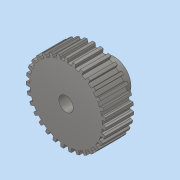
# Autodesk Inventor part: PinionGear
Saved by Autodesk Inventor 2017 (Build 210142000, 142)
## iProperties
Created: 2016-11-06
Part Number: PinionGear
Material: Stainless Steel, Brushed
Document SubType Name: Modeling
Designer: techn
Density: 8 g/cm^3
Appearance: Stainless - Brushed
Author: techn
Comments: 31 Tooth Traxxas Pinion Gear
Autodesk Inventor part; units mm, degrees
ref_plane "YZ Plane" through (0, 0, 0) normal (1, 0, 0) x (0, 1, 0)
ref_plane "XZ Plane" through (0, 0, 0) normal (0, 1, 0) x (-1, 0, 0)
ref_plane "XY Plane" through (0, 0, 0) normal (0, 0, 1) x (1, 0, 0)
sketch "Sketch1" plane through (0, 0, 0) normal (0, 0, 1) x (1, 0, 0)
  circle A0 centre (0, 0) radius 3.7465
  dimension "d0" = 7.493
  constraints: 1 centre point, 1 coincident
  measures "d0" diameter of A0
extrude "Extrusion1" add sketch "Sketch1" along normal blind 10.5156
sketch "Sketch2" plane through (0, 0, 10.5156) normal (0, 0, 1) x (1, 0, 0)
  circle A0 centre (0, 0) radius 8.763
  dimension "d3" = 17.526
  constraints: 1 centre point, 1 coincident
  measures "d3" diameter of A0
extrude "Extrusion2" add sketch "Sketch2" against normal blind 6.096
sketch "Sketch4" plane through (0, 0, 10.5156) normal (0, 0, 1) x (1, 0, 0)
  circle A0 centre (0, 0) radius 1.5875
  dimension "d6" = 3.175
  constraints: 1 centre point, 1 coincident
  measures "d6" diameter of A0
extrude "Extrusion3" cut sketch "Sketch4" against normal through all
sketch "Sketch5" plane through (0, 0, 10.5156) normal (0, 0, 1) x (1, 0, 0)
  circle A0 centre (0, 0) radius 7.9375
  line L0 (0.3683, 7.929) -> (0.3683, 8.31)
  line L1 (0.3683, 8.31) -> (0.2857, 8.89)
  line L2 (0.2857, 8.89) -> (-0.2858, 8.89)
  line L3 (-0.2858, 8.89) -> (-0.3683, 8.31)
  line L4 (-0.3683, 8.31) -> (-0.3683, 7.929)
  line L5 (-0.3683, 7.929) -> (0.3683, 7.929)
  line L6 (-2.0335, 8.0657) -> (-1.9568, 7.6925)
  line L7 (-2.0694, 8.6505) -> (-2.0335, 8.0657)
  line L8 (-1.5096, 8.7655) -> (-2.0694, 8.6505)
  line L9 (-1.312, 8.214) -> (-1.5096, 8.7655)
  line L10 (-1.2353, 7.8408) -> (-1.312, 8.214)
  line L11 (-1.9568, 7.6925) -> (-1.2353, 7.8408)
  line L12 (-3.6155, 7.4913) -> (-3.4653, 7.1411)
  line L13 (-3.7684, 8.0568) -> (-3.6155, 7.4913)
  line L14 (-3.2432, 8.2822) -> (-3.7684, 8.0568)
  line L15 (-2.9386, 7.7817) -> (-3.2432, 8.2822)
  line L16 (-2.7884, 7.4316) -> (-2.9386, 7.7817)
  line L17 (-3.4653, 7.1411) -> (-2.7884, 7.4316)
  line L18 (-5.0495, 6.6101) -> (-4.8318, 6.2974)
  line L19 (-5.3131, 7.1333) -> (-5.0495, 6.6101)
  line L20 (-4.844, 7.4598) -> (-5.3131, 7.1333)
  line L21 (-4.4449, 7.0309) -> (-4.844, 7.4598)
  line L22 (-4.2273, 6.7182) -> (-4.4449, 7.0309)
  line L23 (-4.8318, 6.2974) -> (-4.2273, 6.7182)
  line L24 (-6.2767, 5.4583) -> (-6.0006, 5.1958)
  line L25 (-6.6403, 5.9178) -> (-6.2767, 5.4583)
  line L26 (-6.2465, 6.332) -> (-6.6403, 5.9178)
  line L27 (-5.7692, 5.9922) -> (-6.2465, 6.332)
  line L28 (-5.4931, 5.7297) -> (-5.7692, 5.9922)
  line L29 (-6.0006, 5.1958) -> (-5.4931, 5.7297)
  line L30 (-7.247, 4.0831) -> (-6.9237, 3.8816)
  line L31 (-7.6956, 4.46) -> (-7.247, 4.0831)
  line L32 (-7.3933, 4.945) -> (-7.6956, 4.46)
  line L33 (-6.8574, 4.7082) -> (-7.3933, 4.945)
  line L34 (-6.534, 4.5067) -> (-6.8574, 4.7082)
  line L35 (-6.9237, 3.8816) -> (-6.534, 4.5067)
  line L36 (-7.9206, 2.5407) -> (-7.5633, 2.4084)
  line L37 (-8.4359, 2.8196) -> (-7.9206, 2.5407)
  line L38 (-8.2374, 3.3555) -> (-8.4359, 2.8196)
  line L39 (-7.6648, 3.2315) -> (-8.2374, 3.3555)
  line L40 (-7.3075, 3.0991) -> (-7.6648, 3.2315)
  line L41 (-7.5633, 2.4084) -> (-7.3075, 3.0991)
  line L42 (-8.2699, 0.8943) -> (-7.8933, 0.8366)
  line L43 (-8.8308, 1.0637) -> (-8.2699, 0.8943)
  line L44 (-8.7442, 1.6286) -> (-8.8308, 1.0637)
  line L45 (-8.1584, 1.6224) -> (-8.7442, 1.6286)
  line L46 (-7.7817, 1.5647) -> (-8.1584, 1.6224)
  line L47 (-7.8933, 0.8366) -> (-7.7817, 1.5647)
  line L48 (-8.2806, -0.7887) -> (-7.9001, -0.7694)
  line L49 (-8.8641, -0.7357) -> (-8.2806, -0.7887)
  line L50 (-8.8931, -0.1649) -> (-8.8641, -0.7357)
  line L51 (-8.3179, -0.0531) -> (-8.8931, -0.1649)
  line L52 (-7.9374, -0.0338) -> (-8.3179, -0.0531)
  line L53 (-7.9001, -0.7694) -> (-7.9374, -0.0338)
  line L54 (-7.9524, -2.4395) -> (-7.5835, -2.344)
  line L55 (-8.5346, -2.5049) -> (-7.9524, -2.4395)
  line L56 (-8.6778, -1.9517) -> (-8.5346, -2.5049)
  line L57 (-8.137, -1.7264) -> (-8.6778, -1.9517)
  line L58 (-7.7682, -1.6309) -> (-8.137, -1.7264)
  line L59 (-7.5835, -2.344) -> (-7.7682, -1.6309)
  line L60 (-7.2985, -3.9903) -> (-6.9565, -3.8225)
  line L61 (-7.8556, -4.1717) -> (-7.2985, -3.9903)
  line L62 (-8.1073, -3.6586) -> (-7.8556, -4.1717)
  line L63 (-7.6229, -3.329) -> (-8.1073, -3.6586)
  line L64 (-7.2808, -3.1612) -> (-7.6229, -3.329)
  line L65 (-6.9565, -3.8225) -> (-7.2808, -3.1612)
  line L66 (-6.3459, -5.3778) -> (-6.0446, -5.1446)
  line L67 (-6.8551, -5.6676) -> (-6.3459, -5.3778)
  line L68 (-7.2049, -5.2157) -> (-6.8551, -5.6676)
  line L69 (-6.7967, -4.7953) -> (-7.2049, -5.2157)
  line L70 (-6.4955, -4.5621) -> (-6.7967, -4.7953)
  line L71 (-6.0446, -5.1446) -> (-6.4955, -4.5621)
  line L72 (-5.1334, -6.5451) -> (-4.8852, -6.2561)
  line L73 (-5.5739, -6.9315) -> (-5.1334, -6.5451)
  line L74 (-6.0075, -6.5592) -> (-5.5739, -6.9315)
  line L75 (-5.6923, -6.0653) -> (-6.0075, -6.5592)
  line L76 (-5.4442, -5.7763) -> (-5.6923, -6.0653)
  line L77 (-4.8852, -6.2561) -> (-5.4442, -5.7763)
  line L78 (-3.7108, -7.4445) -> (-3.5259, -7.1114)
  line L79 (-4.0645, -7.9116) -> (-3.7108, -7.4445)
  line L80 (-4.5642, -7.6343) -> (-4.0645, -7.9116)
  line L81 (-4.3549, -7.087) -> (-4.5642, -7.6343)
  line L82 (-4.17, -6.7539) -> (-4.3549, -7.087)
  line L83 (-3.5259, -7.1114) -> (-4.17, -6.7539)
  line L84 (-2.1363, -8.0391) -> (-2.0222, -7.6756)
  line L85 (-2.3887, -8.5678) -> (-2.1363, -8.0391)
  line L86 (-2.934, -8.3968) -> (-2.3887, -8.5678)
  line L87 (-2.8391, -7.8186) -> (-2.934, -8.3968)
  line L88 (-2.725, -7.4551) -> (-2.8391, -7.8186)
  line L89 (-2.0222, -7.6756) -> (-2.725, -7.4551)
  line L90 (-0.4743, -8.3046) -> (-0.4357, -7.9255)
  line L91 (-0.6151, -8.8733) -> (-0.4743, -8.3046)
  line L92 (-1.1837, -8.8155) -> (-0.6151, -8.8733)
  line L93 (-1.2071, -8.2301) -> (-1.1837, -8.8155)
  line L94 (-1.1686, -7.851) -> (-1.2071, -8.2301)
  line L95 (-0.4357, -7.9255) -> (-1.1686, -7.851)
  line L96 (1.2071, -8.2301) -> (1.1686, -7.851)
  line L97 (1.1837, -8.8155) -> (1.2071, -8.2301)
  line L98 (0.6151, -8.8733) -> (1.1837, -8.8155)
  line L99 (0.4743, -8.3046) -> (0.6151, -8.8733)
  line L100 (0.4357, -7.9255) -> (0.4743, -8.3046)
  line L101 (1.1686, -7.851) -> (0.4357, -7.9255)
  line L102 (2.8391, -7.8186) -> (2.725, -7.4551)
  line L103 (2.934, -8.3968) -> (2.8391, -7.8186)
  line L104 (2.3887, -8.5678) -> (2.934, -8.3968)
  line L105 (2.1363, -8.0391) -> (2.3887, -8.5678)
  line L106 (2.0222, -7.6756) -> (2.1363, -8.0391)
  line L107 (2.725, -7.4551) -> (2.0222, -7.6756)
  line L108 (4.3549, -7.087) -> (4.17, -6.7539)
  line L109 (4.5642, -7.6343) -> (4.3549, -7.087)
  line L110 (4.0645, -7.9116) -> (4.5642, -7.6343)
  line L111 (3.7108, -7.4445) -> (4.0645, -7.9116)
  line L112 (3.5259, -7.1114) -> (3.7108, -7.4445)
  line L113 (4.17, -6.7539) -> (3.5259, -7.1114)
  line L114 (5.6923, -6.0653) -> (5.4442, -5.7763)
  line L115 (6.0075, -6.5592) -> (5.6923, -6.0653)
  line L116 (5.5739, -6.9315) -> (6.0075, -6.5592)
  line L117 (5.1334, -6.5451) -> (5.5739, -6.9315)
  line L118 (4.8852, -6.2561) -> (5.1334, -6.5451)
  line L119 (5.4442, -5.7763) -> (4.8852, -6.2561)
  line L120 (6.7967, -4.7953) -> (6.4955, -4.5621)
  line L121 (7.2049, -5.2157) -> (6.7967, -4.7953)
  line L122 (6.8551, -5.6676) -> (7.2049, -5.2157)
  line L123 (6.3459, -5.3778) -> (6.8551, -5.6676)
  line L124 (6.0446, -5.1446) -> (6.3459, -5.3778)
  line L125 (6.4955, -4.5621) -> (6.0446, -5.1446)
  line L126 (7.6229, -3.329) -> (7.2808, -3.1612)
  line L127 (8.1073, -3.6586) -> (7.6229, -3.329)
  line L128 (7.8556, -4.1717) -> (8.1073, -3.6586)
  line L129 (7.2985, -3.9903) -> (7.8556, -4.1717)
  line L130 (6.9565, -3.8225) -> (7.2985, -3.9903)
  line L131 (7.2808, -3.1612) -> (6.9565, -3.8225)
  line L132 (8.137, -1.7264) -> (7.7682, -1.6309)
  line L133 (8.6778, -1.9517) -> (8.137, -1.7264)
  line L134 (8.5346, -2.5049) -> (8.6778, -1.9517)
  line L135 (7.9524, -2.4395) -> (8.5346, -2.5049)
  line L136 (7.5835, -2.344) -> (7.9524, -2.4395)
  line L137 (7.7682, -1.6309) -> (7.5835, -2.344)
  line L138 (8.3179, -0.0531) -> (7.9374, -0.0338)
  line L139 (8.8931, -0.1649) -> (8.3179, -0.0531)
  line L140 (8.8641, -0.7357) -> (8.8931, -0.1649)
  line L141 (8.2806, -0.7887) -> (8.8641, -0.7357)
  line L142 (7.9001, -0.7694) -> (8.2806, -0.7887)
  line L143 (7.9374, -0.0338) -> (7.9001, -0.7694)
  line L144 (8.1584, 1.6224) -> (7.7817, 1.5647)
  line L145 (8.7442, 1.6286) -> (8.1584, 1.6224)
  line L146 (8.8308, 1.0637) -> (8.7442, 1.6286)
  line L147 (8.2699, 0.8943) -> (8.8308, 1.0637)
  line L148 (7.8933, 0.8366) -> (8.2699, 0.8943)
  line L149 (7.7817, 1.5647) -> (7.8933, 0.8366)
  line L150 (7.6648, 3.2315) -> (7.3075, 3.0991)
  line L151 (8.2374, 3.3555) -> (7.6648, 3.2315)
  line L152 (8.4359, 2.8196) -> (8.2374, 3.3555)
  line L153 (7.9206, 2.5407) -> (8.4359, 2.8196)
  line L154 (7.5633, 2.4084) -> (7.9206, 2.5407)
  line L155 (7.3075, 3.0991) -> (7.5633, 2.4084)
  line L156 (6.8574, 4.7082) -> (6.534, 4.5067)
  line L157 (7.3933, 4.945) -> (6.8574, 4.7082)
  line L158 (7.6956, 4.46) -> (7.3933, 4.945)
  line L159 (7.247, 4.0831) -> (7.6956, 4.46)
  line L160 (6.9237, 3.8816) -> (7.247, 4.0831)
  line L161 (6.534, 4.5067) -> (6.9237, 3.8816)
  line L162 (5.7692, 5.9922) -> (5.4931, 5.7297)
  line L163 (6.2465, 6.332) -> (5.7692, 5.9922)
  line L164 (6.6403, 5.9178) -> (6.2465, 6.332)
  line L165 (6.2767, 5.4583) -> (6.6403, 5.9178)
  line L166 (6.0006, 5.1958) -> (6.2767, 5.4583)
  line L167 (5.4931, 5.7297) -> (6.0006, 5.1958)
  line L168 (4.4449, 7.0309) -> (4.2273, 6.7182)
  line L169 (4.844, 7.4598) -> (4.4449, 7.0309)
  line L170 (5.3131, 7.1333) -> (4.844, 7.4598)
  line L171 (5.0495, 6.6101) -> (5.3131, 7.1333)
  line L172 (4.8318, 6.2974) -> (5.0495, 6.6101)
  line L173 (4.2273, 6.7182) -> (4.8318, 6.2974)
  line L174 (2.9386, 7.7817) -> (2.7884, 7.4316)
  line L175 (3.2432, 8.2822) -> (2.9386, 7.7817)
  line L176 (3.7684, 8.0568) -> (3.2432, 8.2822)
  line L177 (3.6155, 7.4913) -> (3.7684, 8.0568)
  line L178 (3.4653, 7.1411) -> (3.6155, 7.4913)
  line L179 (2.7884, 7.4316) -> (3.4653, 7.1411)
  line L180 (1.312, 8.214) -> (1.2353, 7.8408)
  line L181 (1.5096, 8.7655) -> (1.312, 8.214)
  line L182 (2.0694, 8.6505) -> (1.5096, 8.7655)
  line L183 (2.0335, 8.0657) -> (2.0694, 8.6505)
  line L184 (1.9568, 7.6925) -> (2.0335, 8.0657)
  line L185 (1.2353, 7.8408) -> (1.9568, 7.6925)
  circle A1 centre (0, 0) radius 10.3173
  dimension "d9" = 15.875
  dimension "d12" = 360
  dimension "d14" = 0.381
  dimension "d15" = 0.5715
  dimension "d16" = 0.7366
  dimension "d17" = 0.961
  dimension "d18" = 8.89
  constraints: 372 end point, 2 centre point, 2 coincident, 2 equal length, 2 horizontal, 2 point on circle, 1 perpendicular, 1 vertical, 373 other
  measures "d9" diameter of A0
  measures "d14" distance of L0.start L0.end
  measures "d15" distance of L1.end L2.end
  measures "d16" distance of L4.end L0.start
  measures "d17" distance between parallel lines of L2 L5
  measures "d18" distance from line of point (0, 0) L2
extrude "Extrusion4" cut sketch "Sketch5" against normal up to surface (6.096 mm away)
sketch "Sketch6" plane through (0, 0, 4.4196) normal (0, 0, -1) x (-1, 0, 0)
  line L0 (-4.6588, 6.2294) -> (7.7624, 6.2294) construction
  line L1 (7.7624, 6.2294) -> (7.7624, 4.7867) construction
  line L2 (7.7624, 4.7867) -> (-4.6588, 4.7867) construction
  line L3 (-4.6588, 4.7867) -> (-4.6588, 6.2294) construction
  spline S0 degree 2 poles (-4.0162, 6.0091) (-4.0846, 6.0091) (-4.2198, 5.9757) (-4.2851, 5.9499) knots 0 0 0 1 2 2 2
  spline S1 degree 2 poles (-4.2851, 5.9499) (-4.3458, 5.9241) (-4.4355, 5.8694) (-4.4704, 5.8451) knots 0 0 0 1 2 2 2
  line L4 (-4.4704, 5.8451) -> (-4.4856, 5.8451)
  line L5 (-4.4856, 5.8451) -> (-4.4856, 6.1109)
  spline S2 degree 2 poles (-4.4856, 6.1109) (-4.4036, 6.155) (-4.1225, 6.2264) (-3.9965, 6.2264) knots 0 0 0 1 2 2 2
  spline S3 degree 2 poles (-3.9965, 6.2264) (-3.8689, 6.2264) (-3.679, 6.1747) (-3.6015, 6.12) knots 0 0 0 1 2 2 2
  spline S4 degree 2 poles (-3.6015, 6.12) (-3.5195, 6.0608) (-3.4344, 5.8891) (-3.4344, 5.7737) knots 0 0 0 1 2 2 2
  spline S5 degree 2 poles (-3.4344, 5.7737) (-3.4344, 5.6187) (-3.638, 5.3848) (-3.7807, 5.3544) knots 0 0 0 1 2 2 2
  line L6 (-3.7807, 5.3544) -> (-3.7807, 5.3362)
  spline S6 degree 2 poles (-3.7807, 5.3362) (-3.7215, 5.324) (-3.5863, 5.2693) (-3.5286, 5.2147) knots 0 0 0 1 2 2 2
  spline S7 degree 2 poles (-3.5286, 5.2147) (-3.4709, 5.1615) (-3.3979, 4.9914) (-3.3979, 4.8683) knots 0 0 0 1 2 2 2
  spline S8 degree 2 poles (-3.3979, 4.8683) (-3.3979, 4.7422) (-3.4845, 4.528) (-3.5635, 4.446) knots 0 0 0 1 2 2 2
  spline S9 degree 2 poles (-3.5635, 4.446) (-3.6455, 4.3609) (-3.878, 4.2728) (-4.0253, 4.2728) knots 0 0 0 1 2 2 2
  spline S10 degree 2 poles (-4.0253, 4.2728) (-4.1666, 4.2728) (-4.4431, 4.3412) (-4.5372, 4.3883) knots 0 0 0 1 2 2 2
  line L7 (-4.5372, 4.3883) -> (-4.5372, 4.6541)
  line L8 (-4.5372, 4.6541) -> (-4.519, 4.6541)
  spline S11 degree 2 poles (-4.519, 4.6541) (-4.44, 4.5964) (-4.1727, 4.4901) (-4.0405, 4.4901) knots 0 0 0 1 2 2 2
  spline S12 degree 2 poles (-4.0405, 4.4901) (-3.963, 4.4901) (-3.8081, 4.5387) (-3.7564, 4.5949) knots 0 0 0 1 2 2 2
  spline S13 degree 2 poles (-3.7564, 4.5949) (-3.7063, 4.6511) (-3.6531, 4.7848) (-3.6531, 4.8865) knots 0 0 0 1 2 2 2
  spline S14 degree 2 poles (-3.6531, 4.8865) (-3.6531, 4.9883) (-3.7124, 5.1205) (-3.7656, 5.1585) knots 0 0 0 1 2 2 2
  spline S15 degree 2 poles (-3.7656, 5.1585) (-3.8187, 5.1964) (-3.963, 5.2253) (-4.0481, 5.2253) knots 0 0 0 1 2 2 2
  line L9 (-4.0481, 5.2253) -> (-4.1544, 5.2253)
  line L10 (-4.1544, 5.2253) -> (-4.1544, 5.4334)
  line L11 (-4.1544, 5.4334) -> (-4.0709, 5.4334)
  spline S16 degree 2 poles (-4.0709, 5.4334) (-3.9023, 5.4334) (-3.6896, 5.5944) (-3.6896, 5.7478) knots 0 0 0 1 2 2 2
  spline S17 degree 2 poles (-3.6896, 5.7478) (-3.6896, 5.8192) (-3.7443, 5.921) (-3.7883, 5.9514) knots 0 0 0 1 2 2 2
  spline S18 degree 2 poles (-3.7883, 5.9514) (-3.8354, 5.9833) (-3.9509, 6.0091) (-4.0162, 6.0091) knots 0 0 0 1 2 2 2
  line L12 (-2.0536, 4.3123) -> (-2.968, 4.3123)
  line L13 (-2.968, 4.3123) -> (-2.968, 4.5037)
  line L14 (-2.968, 4.5037) -> (-2.6278, 4.5037)
  line L15 (-2.6278, 4.5037) -> (-2.6278, 5.76)
  line L16 (-2.6278, 5.76) -> (-2.968, 5.76)
  line L17 (-2.968, 5.76) -> (-2.968, 5.9317)
  spline S19 degree 2 poles (-2.968, 5.9317) (-2.7751, 5.9317) (-2.5928, 6.041) (-2.5807, 6.1929) knots 0 0 0 1 2 2 2
  line L18 (-2.5807, 6.1929) -> (-2.3862, 6.1929)
  line L19 (-2.3862, 6.1929) -> (-2.3862, 4.5037)
  line L20 (-2.3862, 4.5037) -> (-2.0536, 4.5037)
  line L21 (-2.0536, 4.5037) -> (-2.0536, 4.3123)
  line L22 (-1.2181, 4.3123) -> (-1.2181, 5.9651)
  line L23 (-1.2181, 5.9651) -> (-1.847, 5.9651)
  line L24 (-1.847, 5.9651) -> (-1.847, 6.1869)
  line L25 (-1.847, 6.1869) -> (-0.3401, 6.1869)
  line L26 (-0.3401, 6.1869) -> (-0.3401, 5.9651)
  line L27 (-0.3401, 5.9651) -> (-0.969, 5.9651)
  line L28 (-0.969, 5.9651) -> (-0.969, 4.3123)
  line L29 (-0.969, 4.3123) -> (-1.2181, 4.3123)
  line L30 (1.8079, 4.9564) -> (1.5846, 4.9564)
  line L31 (1.5846, 4.9564) -> (1.5846, 4.3123)
  line L32 (1.5846, 4.3123) -> (1.343, 4.3123)
  line L33 (1.343, 4.3123) -> (1.343, 4.9564)
  line L34 (1.343, 4.9564) -> (0.5152, 4.9564)
  line L35 (0.5152, 4.9564) -> (0.5152, 5.2207)
  line L36 (0.5152, 5.2207) -> (1.3537, 6.1869)
  line L37 (1.3537, 6.1869) -> (1.5846, 6.1869)
  line L38 (1.5846, 6.1869) -> (1.5846, 5.1585)
  line L39 (1.5846, 5.1585) -> (1.8079, 5.1585)
  line L40 (1.8079, 5.1585) -> (1.8079, 4.9564)
  line L41 (1.343, 5.1585) -> (1.343, 5.8906)
  line L42 (1.343, 5.8906) -> (0.7126, 5.1585)
  line L43 (0.7126, 5.1585) -> (1.343, 5.1585)
  spline S20 degree 2 poles (2.575, 4.2698) (2.4352, 4.2698) (2.2059, 4.3534) (2.1254, 4.4308) knots 0 0 0 1 2 2 2
  spline S21 degree 2 poles (2.1254, 4.4308) (2.0464, 4.5068) (1.9643, 4.7134) (1.9643, 4.8303) knots 0 0 0 1 2 2 2
  spline S22 degree 2 poles (1.9643, 4.8303) (1.9643, 4.9822) (2.1269, 5.2374) (2.2818, 5.3134) knots 0 0 0 1 2 2 2
  line L44 (2.2818, 5.3134) -> (2.2818, 5.321)
  spline S23 degree 2 poles (2.2818, 5.321) (2.1436, 5.4015) (2.0099, 5.5929) (2.0099, 5.7357) knots 0 0 0 1 2 2 2
  spline S24 degree 2 poles (2.0099, 5.7357) (2.0099, 5.9468) (2.3289, 6.2294) (2.575, 6.2294) knots 0 0 0 1 2 2 2
  spline S25 degree 2 poles (2.575, 6.2294) (2.8302, 6.2294) (3.1386, 5.962) (3.1386, 5.7524) knots 0 0 0 1 2 2 2
  spline S26 degree 2 poles (3.1386, 5.7524) (3.1386, 5.6263) (2.9912, 5.3802) (2.853, 5.3104) knots 0 0 0 1 2 2 2
  line L45 (2.853, 5.3104) -> (2.853, 5.3028)
  spline S27 degree 2 poles (2.853, 5.3028) (3.017, 5.2268) (3.1857, 5.0081) (3.1857, 4.8349) knots 0 0 0 1 2 2 2
  spline S28 degree 2 poles (3.1857, 4.8349) (3.1857, 4.5949) (2.8363, 4.2698) (2.575, 4.2698) knots 0 0 0 1 2 2 2
  spline S29 degree 2 poles (2.9274, 4.8106) (2.9274, 4.926) (2.8363, 5.0628) (2.7072, 5.1326) knots 0 0 0 1 2 2 2
  spline S30 degree 2 poles (2.7072, 5.1326) (2.6646, 5.1569) (2.5218, 5.2131) (2.4322, 5.2496) knots 0 0 0 1 2 2 2
  spline S31 degree 2 poles (2.4322, 5.2496) (2.3289, 5.1812) (2.218, 4.9777) (2.218, 4.8486) knots 0 0 0 1 2 2 2
  spline S32 degree 2 poles (2.218, 4.8486) (2.218, 4.6784) (2.4231, 4.4566) (2.578, 4.4566) knots 0 0 0 1 2 2 2
  spline S33 degree 2 poles (2.578, 4.4566) (2.736, 4.4566) (2.9274, 4.6465) (2.9274, 4.8106) knots 0 0 0 1 2 2 2
  spline S34 degree 2 poles (2.8925, 5.7494) (2.8925, 5.8754) (2.7239, 6.0441) (2.5735, 6.0441) knots 0 0 0 1 2 2 2
  spline S35 degree 2 poles (2.5735, 6.0441) (2.4368, 6.0441) (2.2621, 5.8937) (2.2621, 5.7646) knots 0 0 0 1 2 2 2
  spline S36 degree 2 poles (2.2621, 5.7646) (2.2621, 5.6719) (2.3517, 5.5428) (2.4413, 5.4911) knots 0 0 0 1 2 2 2
  spline S37 degree 2 poles (2.4413, 5.4911) (2.4793, 5.4699) (2.6403, 5.3954) (2.7056, 5.3742) knots 0 0 0 1 2 2 2
  spline S38 degree 2 poles (2.7056, 5.3742) (2.815, 5.4577) (2.8925, 5.6354) (2.8925, 5.7494) knots 0 0 0 1 2 2 2
  spline S39 degree 2 poles (4.6531, 5.6218) (4.6531, 5.5002) (4.5665, 5.2815) (4.489, 5.2055) knots 0 0 0 1 2 2 2
  spline S40 degree 2 poles (4.489, 5.2055) (4.3918, 5.1098) (4.129, 5.0111) (3.9285, 5.0111) knots 0 0 0 1 2 2 2
  line L46 (3.9285, 5.0111) -> (3.7173, 5.0111)
  line L47 (3.7173, 5.0111) -> (3.7173, 4.3123)
  line L48 (3.7173, 4.3123) -> (3.4682, 4.3123)
  line L49 (3.4682, 4.3123) -> (3.4682, 6.1869)
  line L50 (3.4682, 6.1869) -> (3.9391, 6.1869)
  spline S41 degree 2 poles (3.9391, 6.1869) (4.1062, 6.1869) (4.3402, 6.1322) (4.4298, 6.0699) knots 0 0 0 1 2 2 2
  spline S42 degree 2 poles (4.4298, 6.0699) (4.5346, 5.9985) (4.6531, 5.7782) (4.6531, 5.6218) knots 0 0 0 1 2 2 2
  spline S43 degree 2 poles (4.3933, 5.6142) (4.3933, 5.7114) (4.3265, 5.8542) (4.2581, 5.8998) knots 0 0 0 1 2 2 2
  spline S44 degree 2 poles (4.2581, 5.8998) (4.1989, 5.9392) (4.0409, 5.9712) (3.9239, 5.9712) knots 0 0 0 1 2 2 2
  line L51 (3.9239, 5.9712) -> (3.7173, 5.9712)
  line L52 (3.7173, 5.9712) -> (3.7173, 5.2238)
  line L53 (3.7173, 5.2238) -> (3.8875, 5.2238)
  spline S45 degree 2 poles (3.8875, 5.2238) (4.0394, 5.2238) (4.2262, 5.2724) (4.287, 5.3362) knots 0 0 0 1 2 2 2
  spline S46 degree 2 poles (4.287, 5.3362) (4.3432, 5.3924) (4.3933, 5.5245) (4.3933, 5.6142) knots 0 0 0 1 2 2 2
  point P0 (0, 0)
  constraints: 2 other
emboss "Emboss1" sketch "Sketch6" operation cut depth 0.254 direction (0, 0, 1)
body "Solid1"
